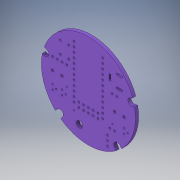
# Autodesk Inventor part: PCB
Saved by Autodesk Inventor 2018 (Build 220112000, 112)
## iProperties
Created: 2017-04-09
Part Number: PCB
Material: Fiberglass Batt
Document SubType Name: Modeling
Designer: dktur
Density: 0.032 g/cm^3
Appearance: Violet
Author: dktur
Autodesk Inventor part; units mm, degrees
ref_plane "YZ Plane" through (0, 0, 0) normal (1, 0, 0) x (0, 1, 0)
ref_plane "XZ Plane" through (0, 0, 0) normal (0, 1, 0) x (-1, 0, 0)
ref_plane "XY Plane" through (0, 0, 0) normal (0, 0, 1) x (1, 0, 0)
sketch "Sketch1" plane through (0, 0, 0) normal (0, 0, 1) x (1, 0, 0)
  arc A0 (14.5033, 41.5512) -> (15.7358, 44.915) centre (15.225, 43.1944) ccw
  line L0 (15.7358, 44.915) -> (14.5707, 45.3269)
  line L1 (14.5033, 41.5512) -> (13.575, 41.9589)
  arc A1 (24.2884, 17.9351) -> (21.5624, 20.3195) centre (22.9253, 19.1272) ccw
  line L2 (21.5624, 20.3195) -> (20.4482, 19.1255)
  line L3 (24.2884, 17.9351) -> (23.3266, 16.7167)
  arc A2 (60.3359, 44.8761) -> (61.4886, 41.4217) centre (60.8858, 43.1401) ccw
  line L4 (60.3359, 44.8761) -> (61.599, 45.4156)
  line L5 (61.4886, 41.4217) -> (62.5849, 41.742)
  arc A3 (54.5374, 20.4215) -> (51.9475, 17.877) centre (53.3634, 19.0261) ccw
  line L6 (51.9475, 17.877) -> (52.8261, 16.6745)
  line L7 (54.5374, 20.4215) -> (55.7157, 19.0618)
  arc A4 (61.599, 45.4156) -> (14.5707, 45.3269) centre (38.1009, 36.8543) ccw
  arc A5 (55.7157, 19.0618) -> (62.5849, 41.742) centre (38.1082, 36.775) ccw
  arc A6 (23.3266, 16.7167) -> (52.8261, 16.6745) centre (38.1052, 36.8421) ccw
  arc A7 (13.575, 41.9589) -> (20.4482, 19.1255) centre (38.0481, 36.8745) ccw
  circle A8 centre (33.274, 19.05) radius 1.651
  circle A9 centre (52.07, 34.29) radius 0.65
  circle A10 centre (57.07, 34.29) radius 0.65
  circle A11 centre (48.26, 19.05) radius 0.508
  circle A12 centre (48.26, 16.51) radius 0.508
  circle A13 centre (48.26, 21.59) radius 0.508
  circle A14 centre (52.07, 25.4) radius 0.508
  circle A15 centre (49.53, 25.4) radius 0.508
  circle A16 centre (45.72, 48.26) radius 0.508
  circle A17 centre (45.72, 50.8) radius 0.508
  circle A18 centre (45.72, 53.34) radius 0.508
  circle A19 centre (45.72, 55.88) radius 0.508
  circle A20 centre (19.05, 30.48) radius 0.4064
  circle A21 centre (20.955, 29.21) radius 0.4064
  circle A22 centre (19.05, 27.94) radius 0.4064
  circle A23 centre (19.05, 36.83) radius 0.65
  circle A24 centre (24.05, 36.83) radius 0.65
  circle A25 centre (30.48, 24.13) radius 0.3
  circle A26 centre (50.8, 27.94) radius 0.3
  circle A27 centre (26.67, 33.02) radius 0.3
  circle A28 centre (54.57, 52.19) radius 0.5
  circle A29 centre (49.57, 48.89) radius 0.5
  circle A30 centre (54.57, 45.89) radius 0.5
  circle A31 centre (53.34, 41.91) radius 0.508
  circle A32 centre (50.8, 41.91) radius 0.508
  circle A33 centre (33.02, 29.21) radius 0.508
  circle A34 centre (57.15, 29.21) radius 0.4064
  circle A35 centre (59.055, 27.94) radius 0.4064
  circle A36 centre (57.15, 26.67) radius 0.4064
  circle A37 centre (19.05, 43.18) radius 0.508
  circle A38 centre (21.59, 43.18) radius 0.508
  circle A39 centre (24.13, 43.18) radius 0.508
  circle A40 centre (26.67, 43.18) radius 0.508
  circle A41 centre (24.13, 30.48) radius 0.4064
  circle A42 centre (26.035, 29.21) radius 0.4064
  circle A43 centre (24.13, 27.94) radius 0.4064
  circle A44 centre (27.6606, 46.2788) radius 0.508
  circle A45 centre (27.6606, 52.7812) radius 0.508
  circle A46 centre (23.1394, 46.2788) radius 0.508
  circle A47 centre (23.1394, 52.7812) radius 0.508
  circle A48 centre (30.48, 55.88) radius 0.508
  circle A49 centre (30.48, 53.34) radius 0.508
  circle A50 centre (30.48, 50.8) radius 0.508
  circle A51 centre (30.48, 48.26) radius 0.508
  circle A52 centre (30.48, 45.72) radius 0.508
  circle A53 centre (30.48, 43.18) radius 0.508
  circle A54 centre (30.48, 40.64) radius 0.508
  circle A55 centre (30.48, 38.1) radius 0.508
  circle A56 centre (30.48, 35.56) radius 0.508
  circle A57 centre (30.48, 33.02) radius 0.508
  circle A58 centre (30.48, 30.48) radius 0.508
  circle A59 centre (30.48, 27.94) radius 0.508
  circle A60 centre (45.72, 27.94) radius 0.508
  circle A61 centre (45.72, 30.48) radius 0.508
  circle A62 centre (45.72, 33.02) radius 0.508
  circle A63 centre (45.72, 35.56) radius 0.508
  circle A64 centre (45.72, 38.1) radius 0.508
  circle A65 centre (45.72, 40.64) radius 0.508
  circle A66 centre (45.72, 43.18) radius 0.508
  circle A67 centre (45.72, 45.72) radius 0.508
  line L8 (56.17, 45.89) -> (52.97, 45.89)
  arc A68 (55.67, 45.39) -> (56.17, 45.89) centre (55.67, 45.89) ccw
  line L9 (55.67, 45.39) -> (53.47, 45.39)
  arc A69 (52.97, 45.89) -> (53.47, 45.39) centre (53.47, 45.89) ccw
  arc A70 (53.47, 46.39) -> (52.97, 45.89) centre (53.47, 45.89) ccw
  line L10 (53.47, 46.39) -> (55.67, 46.39)
  arc A71 (56.17, 45.89) -> (55.67, 46.39) centre (55.67, 45.89) ccw
  arc A72 (55.67, 51.69) -> (56.17, 52.19) centre (55.67, 52.19) ccw
  line L11 (55.67, 51.69) -> (53.47, 51.69)
  arc A73 (52.97, 52.19) -> (53.47, 51.69) centre (53.47, 52.19) ccw
  arc A74 (53.47, 52.69) -> (52.97, 52.19) centre (53.47, 52.19) ccw
  line L12 (53.47, 52.69) -> (55.67, 52.69)
  arc A75 (49.57, 47.29) -> (50.07, 47.79) centre (49.57, 47.79) ccw
  arc A76 (49.07, 47.79) -> (49.57, 47.29) centre (49.57, 47.79) ccw
  line L13 (49.07, 47.79) -> (49.07, 49.99)
  arc A77 (49.57, 50.49) -> (49.07, 49.99) centre (49.57, 49.99) ccw
  arc A78 (50.07, 49.99) -> (49.57, 50.49) centre (49.57, 49.99) ccw
  arc A79 (56.17, 52.19) -> (55.67, 52.69) centre (55.67, 52.19) ccw
  line L14 (50.07, 49.99) -> (50.07, 47.79)
  arc A80 (57.07, 33.782) -> (57.07, 34.798) centre (57.07, 34.29) ccw
  arc A81 (57.07, 34.798) -> (57.07, 33.782) centre (57.07, 34.29) ccw
  arc A82 (57.07, 33.782) -> (57.07, 34.798) centre (57.07, 34.29) ccw
  arc A83 (57.07, 34.798) -> (57.07, 33.782) centre (57.07, 34.29) ccw
  line L15 (49.022, 19.05) -> (47.498, 19.05)
  arc A84 (47.498, 19.431) -> (47.498, 18.669) centre (47.498, 19.05) ccw
  arc A85 (49.022, 18.669) -> (49.022, 19.431) centre (49.022, 19.05) ccw
  line L16 (49.022, 19.05) -> (47.498, 19.05)
  arc A86 (47.498, 19.431) -> (47.498, 18.669) centre (47.498, 19.05) ccw
  arc A87 (49.022, 18.669) -> (49.022, 19.431) centre (49.022, 19.05) ccw
  line L17 (49.022, 16.51) -> (47.498, 16.51)
  arc A88 (47.498, 16.891) -> (47.498, 16.129) centre (47.498, 16.51) ccw
  arc A89 (49.022, 16.129) -> (49.022, 16.891) centre (49.022, 16.51) ccw
  line L18 (49.022, 16.51) -> (47.498, 16.51)
  arc A90 (47.498, 16.891) -> (47.498, 16.129) centre (47.498, 16.51) ccw
  arc A91 (49.022, 16.129) -> (49.022, 16.891) centre (49.022, 16.51) ccw
  line L19 (49.022, 21.59) -> (47.498, 21.59)
  arc A92 (47.498, 21.971) -> (47.498, 21.209) centre (47.498, 21.59) ccw
  arc A93 (49.022, 21.209) -> (49.022, 21.971) centre (49.022, 21.59) ccw
  line L20 (49.022, 21.59) -> (47.498, 21.59)
  arc A94 (47.498, 21.971) -> (47.498, 21.209) centre (47.498, 21.59) ccw
  arc A95 (49.022, 21.209) -> (49.022, 21.971) centre (49.022, 21.59) ccw
  arc A96 (51.6001, 25.4) -> (52.5399, 25.4) centre (52.07, 25.4) ccw
  arc A97 (52.5399, 25.4) -> (51.6001, 25.4) centre (52.07, 25.4) ccw
  arc A98 (51.6001, 25.4) -> (52.5399, 25.4) centre (52.07, 25.4) ccw
  arc A99 (52.5399, 25.4) -> (51.6001, 25.4) centre (52.07, 25.4) ccw
  arc A100 (49.0601, 25.4) -> (49.9999, 25.4) centre (49.53, 25.4) ccw
  arc A101 (49.9999, 25.4) -> (49.0601, 25.4) centre (49.53, 25.4) ccw
  arc A102 (49.0601, 25.4) -> (49.9999, 25.4) centre (49.53, 25.4) ccw
  arc A103 (49.9999, 25.4) -> (49.0601, 25.4) centre (49.53, 25.4) ccw
  line L21 (55.57, 52.19) -> (53.57, 52.19)
  arc A104 (53.57, 52.69) -> (53.57, 51.69) centre (53.57, 52.19) ccw
  arc A105 (55.57, 51.69) -> (55.57, 52.69) centre (55.57, 52.19) ccw
  line L22 (55.57, 52.19) -> (53.57, 52.19)
  arc A106 (53.57, 52.69) -> (53.57, 51.69) centre (53.57, 52.19) ccw
  arc A107 (55.57, 51.69) -> (55.57, 52.69) centre (55.57, 52.19) ccw
  line L23 (49.57, 49.89) -> (49.57, 47.89)
  arc A108 (49.07, 47.89) -> (50.07, 47.89) centre (49.57, 47.89) ccw
  arc A109 (50.07, 49.89) -> (49.07, 49.89) centre (49.57, 49.89) ccw
  line L24 (49.57, 49.89) -> (49.57, 47.89)
  arc A110 (49.07, 47.89) -> (50.07, 47.89) centre (49.57, 47.89) ccw
  arc A111 (50.07, 49.89) -> (49.07, 49.89) centre (49.57, 49.89) ccw
  line L25 (55.57, 45.89) -> (53.57, 45.89)
  arc A112 (53.57, 46.39) -> (53.57, 45.39) centre (53.57, 45.89) ccw
  arc A113 (55.57, 45.39) -> (55.57, 46.39) centre (55.57, 45.89) ccw
  line L26 (55.57, 45.89) -> (53.57, 45.89)
  arc A114 (53.57, 46.39) -> (53.57, 45.39) centre (53.57, 45.89) ccw
  arc A115 (55.57, 45.39) -> (55.57, 46.39) centre (55.57, 45.89) ccw
  arc A116 (52.8701, 41.91) -> (53.8099, 41.91) centre (53.34, 41.91) ccw
  arc A117 (53.8099, 41.91) -> (52.8701, 41.91) centre (53.34, 41.91) ccw
  arc A118 (52.8701, 41.91) -> (53.8099, 41.91) centre (53.34, 41.91) ccw
  arc A119 (53.8099, 41.91) -> (52.8701, 41.91) centre (53.34, 41.91) ccw
  arc A120 (50.3301, 41.91) -> (51.2699, 41.91) centre (50.8, 41.91) ccw
  arc A121 (51.2699, 41.91) -> (50.3301, 41.91) centre (50.8, 41.91) ccw
  arc A122 (50.3301, 41.91) -> (51.2699, 41.91) centre (50.8, 41.91) ccw
  arc A123 (51.2699, 41.91) -> (50.3301, 41.91) centre (50.8, 41.91) ccw
  line L27 (57.2763, 28.9052) -> (57.0237, 28.9052)
  line L28 (57.0237, 28.9052) -> (56.8452, 29.0837)
  line L29 (56.8452, 29.0837) -> (56.8452, 29.3363)
  line L30 (56.8452, 29.3363) -> (57.0237, 29.5148)
  line L31 (57.0237, 29.5148) -> (57.2763, 29.5148)
  line L32 (57.2763, 29.5148) -> (57.4548, 29.3363)
  line L33 (57.4548, 29.3363) -> (57.4548, 29.0837)
  line L34 (57.4548, 29.0837) -> (57.2763, 28.9052)
  line L35 (57.2763, 28.9052) -> (57.0237, 28.9052)
  line L36 (57.2763, 28.9052) -> (57.0237, 28.9052)
  line L37 (57.0237, 28.9052) -> (56.8452, 29.0837)
  line L38 (56.8452, 29.0837) -> (56.8452, 29.3363)
  line L39 (56.8452, 29.3363) -> (57.0237, 29.5148)
  line L40 (57.0237, 29.5148) -> (57.2763, 29.5148)
  line L41 (57.2763, 29.5148) -> (57.4548, 29.3363)
  line L42 (57.4548, 29.3363) -> (57.4548, 29.0837)
  line L43 (57.4548, 29.0837) -> (57.2763, 28.9052)
  line L44 (57.2763, 28.9052) -> (57.0237, 28.9052)
  line L45 (59.1813, 27.6352) -> (58.9287, 27.6352)
  line L46 (58.9287, 27.6352) -> (58.7502, 27.8137)
  line L47 (58.7502, 27.8137) -> (58.7502, 28.0663)
  line L48 (58.7502, 28.0663) -> (58.9287, 28.2448)
  line L49 (58.9287, 28.2448) -> (59.1813, 28.2448)
  line L50 (59.1813, 28.2448) -> (59.3598, 28.0663)
  line L51 (59.3598, 28.0663) -> (59.3598, 27.8137)
  line L52 (59.3598, 27.8137) -> (59.1813, 27.6352)
  line L53 (59.1813, 27.6352) -> (58.9287, 27.6352)
  line L54 (59.1813, 27.6352) -> (58.9287, 27.6352)
  line L55 (58.9287, 27.6352) -> (58.7502, 27.8137)
  line L56 (58.7502, 27.8137) -> (58.7502, 28.0663)
  line L57 (58.7502, 28.0663) -> (58.9287, 28.2448)
  line L58 (58.9287, 28.2448) -> (59.1813, 28.2448)
  line L59 (59.1813, 28.2448) -> (59.3598, 28.0663)
  line L60 (59.3598, 28.0663) -> (59.3598, 27.8137)
  line L61 (59.3598, 27.8137) -> (59.1813, 27.6352)
  line L62 (59.1813, 27.6352) -> (58.9287, 27.6352)
  line L63 (57.2763, 26.3652) -> (57.0237, 26.3652)
  line L64 (57.0237, 26.3652) -> (56.8452, 26.5437)
  line L65 (56.8452, 26.5437) -> (56.8452, 26.7963)
  line L66 (56.8452, 26.7963) -> (57.0237, 26.9748)
  line L67 (57.0237, 26.9748) -> (57.2763, 26.9748)
  line L68 (57.2763, 26.9748) -> (57.4548, 26.7963)
  line L69 (57.4548, 26.7963) -> (57.4548, 26.5437)
  line L70 (57.4548, 26.5437) -> (57.2763, 26.3652)
  line L71 (57.2763, 26.3652) -> (57.0237, 26.3652)
  line L72 (57.2763, 26.3652) -> (57.0237, 26.3652)
  line L73 (57.0237, 26.3652) -> (56.8452, 26.5437)
  line L74 (56.8452, 26.5437) -> (56.8452, 26.7963)
  line L75 (56.8452, 26.7963) -> (57.0237, 26.9748)
  line L76 (57.0237, 26.9748) -> (57.2763, 26.9748)
  line L77 (57.2763, 26.9748) -> (57.4548, 26.7963)
  line L78 (57.4548, 26.7963) -> (57.4548, 26.5437)
  line L79 (57.4548, 26.5437) -> (57.2763, 26.3652)
  line L80 (57.2763, 26.3652) -> (57.0237, 26.3652)
  arc A124 (19.5199, 43.18) -> (18.5801, 43.18) centre (19.05, 43.18) ccw
  arc A125 (18.5801, 43.18) -> (19.5199, 43.18) centre (19.05, 43.18) ccw
  arc A126 (19.5199, 43.18) -> (18.5801, 43.18) centre (19.05, 43.18) ccw
  arc A127 (18.5801, 43.18) -> (19.5199, 43.18) centre (19.05, 43.18) ccw
  arc A128 (22.0599, 43.18) -> (21.1201, 43.18) centre (21.59, 43.18) ccw
  arc A129 (21.1201, 43.18) -> (22.0599, 43.18) centre (21.59, 43.18) ccw
  arc A130 (22.0599, 43.18) -> (21.1201, 43.18) centre (21.59, 43.18) ccw
  arc A131 (21.1201, 43.18) -> (22.0599, 43.18) centre (21.59, 43.18) ccw
  arc A132 (24.5999, 43.18) -> (23.6601, 43.18) centre (24.13, 43.18) ccw
  arc A133 (23.6601, 43.18) -> (24.5999, 43.18) centre (24.13, 43.18) ccw
  arc A134 (24.5999, 43.18) -> (23.6601, 43.18) centre (24.13, 43.18) ccw
  arc A135 (23.6601, 43.18) -> (24.5999, 43.18) centre (24.13, 43.18) ccw
  arc A136 (27.1399, 43.18) -> (26.2001, 43.18) centre (26.67, 43.18) ccw
  arc A137 (26.2001, 43.18) -> (27.1399, 43.18) centre (26.67, 43.18) ccw
  arc A138 (27.1399, 43.18) -> (26.2001, 43.18) centre (26.67, 43.18) ccw
  arc A139 (26.2001, 43.18) -> (27.1399, 43.18) centre (26.67, 43.18) ccw
  line L81 (24.2563, 30.1752) -> (24.0037, 30.1752)
  line L82 (24.0037, 30.1752) -> (23.8252, 30.3537)
  line L83 (23.8252, 30.3537) -> (23.8252, 30.6063)
  line L84 (23.8252, 30.6063) -> (24.0037, 30.7848)
  line L85 (24.0037, 30.7848) -> (24.2563, 30.7848)
  line L86 (24.2563, 30.7848) -> (24.4348, 30.6063)
  line L87 (24.4348, 30.6063) -> (24.4348, 30.3537)
  line L88 (24.4348, 30.3537) -> (24.2563, 30.1752)
  line L89 (24.2563, 30.1752) -> (24.0037, 30.1752)
  line L90 (24.2563, 30.1752) -> (24.0037, 30.1752)
  line L91 (24.0037, 30.1752) -> (23.8252, 30.3537)
  line L92 (23.8252, 30.3537) -> (23.8252, 30.6063)
  line L93 (23.8252, 30.6063) -> (24.0037, 30.7848)
  line L94 (24.0037, 30.7848) -> (24.2563, 30.7848)
  line L95 (24.2563, 30.7848) -> (24.4348, 30.6063)
  line L96 (24.4348, 30.6063) -> (24.4348, 30.3537)
  line L97 (24.4348, 30.3537) -> (24.2563, 30.1752)
  line L98 (24.2563, 30.1752) -> (24.0037, 30.1752)
  line L99 (26.1613, 28.9052) -> (25.9087, 28.9052)
  line L100 (25.9087, 28.9052) -> (25.7302, 29.0837)
  line L101 (25.7302, 29.0837) -> (25.7302, 29.3363)
  line L102 (25.7302, 29.3363) -> (25.9087, 29.5148)
  line L103 (25.9087, 29.5148) -> (26.1613, 29.5148)
  line L104 (26.1613, 29.5148) -> (26.3398, 29.3363)
  line L105 (26.3398, 29.3363) -> (26.3398, 29.0837)
  line L106 (26.3398, 29.0837) -> (26.1613, 28.9052)
  line L107 (26.1613, 28.9052) -> (25.9087, 28.9052)
  line L108 (26.1613, 28.9052) -> (25.9087, 28.9052)
  line L109 (25.9087, 28.9052) -> (25.7302, 29.0837)
  line L110 (25.7302, 29.0837) -> (25.7302, 29.3363)
  line L111 (25.7302, 29.3363) -> (25.9087, 29.5148)
  line L112 (25.9087, 29.5148) -> (26.1613, 29.5148)
  line L113 (26.1613, 29.5148) -> (26.3398, 29.3363)
  line L114 (26.3398, 29.3363) -> (26.3398, 29.0837)
  line L115 (26.3398, 29.0837) -> (26.1613, 28.9052)
  line L116 (26.1613, 28.9052) -> (25.9087, 28.9052)
  line L117 (24.2563, 27.6352) -> (24.0037, 27.6352)
  line L118 (24.0037, 27.6352) -> (23.8252, 27.8137)
  line L119 (23.8252, 27.8137) -> (23.8252, 28.0663)
  line L120 (23.8252, 28.0663) -> (24.0037, 28.2448)
  line L121 (24.0037, 28.2448) -> (24.2563, 28.2448)
  line L122 (24.2563, 28.2448) -> (24.4348, 28.0663)
  line L123 (24.4348, 28.0663) -> (24.4348, 27.8137)
  line L124 (24.4348, 27.8137) -> (24.2563, 27.6352)
  line L125 (24.2563, 27.6352) -> (24.0037, 27.6352)
  line L126 (24.2563, 27.6352) -> (24.0037, 27.6352)
  line L127 (24.0037, 27.6352) -> (23.8252, 27.8137)
  line L128 (23.8252, 27.8137) -> (23.8252, 28.0663)
  line L129 (23.8252, 28.0663) -> (24.0037, 28.2448)
  line L130 (24.0037, 28.2448) -> (24.2563, 28.2448)
  line L131 (24.2563, 28.2448) -> (24.4348, 28.0663)
  line L132 (24.4348, 28.0663) -> (24.4348, 27.8137)
  line L133 (24.4348, 27.8137) -> (24.2563, 27.6352)
  line L134 (24.2563, 27.6352) -> (24.0037, 27.6352)
  arc A140 (28.1305, 46.2788) -> (27.1907, 46.2788) centre (27.6606, 46.2788) ccw
  arc A141 (27.1907, 46.2788) -> (28.1305, 46.2788) centre (27.6606, 46.2788) ccw
  arc A142 (28.1305, 46.2788) -> (27.1907, 46.2788) centre (27.6606, 46.2788) ccw
  arc A143 (27.1907, 46.2788) -> (28.1305, 46.2788) centre (27.6606, 46.2788) ccw
  arc A144 (28.1305, 52.7812) -> (27.1907, 52.7812) centre (27.6606, 52.7812) ccw
  arc A145 (27.1907, 52.7812) -> (28.1305, 52.7812) centre (27.6606, 52.7812) ccw
  arc A146 (28.1305, 52.7812) -> (27.1907, 52.7812) centre (27.6606, 52.7812) ccw
  arc A147 (27.1907, 52.7812) -> (28.1305, 52.7812) centre (27.6606, 52.7812) ccw
  arc A148 (23.6093, 46.2788) -> (22.6695, 46.2788) centre (23.1394, 46.2788) ccw
  arc A149 (22.6695, 46.2788) -> (23.6093, 46.2788) centre (23.1394, 46.2788) ccw
  arc A150 (23.6093, 46.2788) -> (22.6695, 46.2788) centre (23.1394, 46.2788) ccw
  arc A151 (22.6695, 46.2788) -> (23.6093, 46.2788) centre (23.1394, 46.2788) ccw
  arc A152 (23.6093, 52.7812) -> (22.6695, 52.7812) centre (23.1394, 52.7812) ccw
  arc A153 (22.6695, 52.7812) -> (23.6093, 52.7812) centre (23.1394, 52.7812) ccw
  arc A154 (23.6093, 52.7812) -> (22.6695, 52.7812) centre (23.1394, 52.7812) ccw
  arc A155 (22.6695, 52.7812) -> (23.6093, 52.7812) centre (23.1394, 52.7812) ccw
  arc A156 (30.48, 55.4101) -> (30.48, 56.3499) centre (30.48, 55.88) ccw
  arc A157 (30.48, 56.3499) -> (30.48, 55.4101) centre (30.48, 55.88) ccw
  arc A158 (30.48, 55.4101) -> (30.48, 56.3499) centre (30.48, 55.88) ccw
  arc A159 (30.48, 56.3499) -> (30.48, 55.4101) centre (30.48, 55.88) ccw
  arc A160 (30.48, 52.8701) -> (30.48, 53.8099) centre (30.48, 53.34) ccw
  arc A161 (30.48, 53.8099) -> (30.48, 52.8701) centre (30.48, 53.34) ccw
  arc A162 (30.48, 52.8701) -> (30.48, 53.8099) centre (30.48, 53.34) ccw
  arc A163 (30.48, 53.8099) -> (30.48, 52.8701) centre (30.48, 53.34) ccw
  arc A164 (30.48, 50.3301) -> (30.48, 51.2699) centre (30.48, 50.8) ccw
  arc A165 (30.48, 51.2699) -> (30.48, 50.3301) centre (30.48, 50.8) ccw
  arc A166 (30.48, 50.3301) -> (30.48, 51.2699) centre (30.48, 50.8) ccw
  arc A167 (30.48, 51.2699) -> (30.48, 50.3301) centre (30.48, 50.8) ccw
  arc A168 (30.48, 47.7901) -> (30.48, 48.7299) centre (30.48, 48.26) ccw
  arc A169 (30.48, 48.7299) -> (30.48, 47.7901) centre (30.48, 48.26) ccw
  arc A170 (30.48, 47.7901) -> (30.48, 48.7299) centre (30.48, 48.26) ccw
  arc A171 (30.48, 48.7299) -> (30.48, 47.7901) centre (30.48, 48.26) ccw
  arc A172 (30.48, 45.2501) -> (30.48, 46.1899) centre (30.48, 45.72) ccw
  arc A173 (30.48, 46.1899) -> (30.48, 45.2501) centre (30.48, 45.72) ccw
  arc A174 (30.48, 45.2501) -> (30.48, 46.1899) centre (30.48, 45.72) ccw
  arc A175 (30.48, 46.1899) -> (30.48, 45.2501) centre (30.48, 45.72) ccw
  arc A176 (30.48, 42.7101) -> (30.48, 43.6499) centre (30.48, 43.18) ccw
  arc A177 (30.48, 43.6499) -> (30.48, 42.7101) centre (30.48, 43.18) ccw
  arc A178 (30.48, 42.7101) -> (30.48, 43.6499) centre (30.48, 43.18) ccw
  arc A179 (30.48, 43.6499) -> (30.48, 42.7101) centre (30.48, 43.18) ccw
  arc A180 (30.48, 40.1701) -> (30.48, 41.1099) centre (30.48, 40.64) ccw
  arc A181 (30.48, 41.1099) -> (30.48, 40.1701) centre (30.48, 40.64) ccw
  arc A182 (30.48, 40.1701) -> (30.48, 41.1099) centre (30.48, 40.64) ccw
  arc A183 (30.48, 41.1099) -> (30.48, 40.1701) centre (30.48, 40.64) ccw
  arc A184 (30.48, 37.6301) -> (30.48, 38.5699) centre (30.48, 38.1) ccw
  arc A185 (30.48, 38.5699) -> (30.48, 37.6301) centre (30.48, 38.1) ccw
  arc A186 (30.48, 37.6301) -> (30.48, 38.5699) centre (30.48, 38.1) ccw
  arc A187 (30.48, 38.5699) -> (30.48, 37.6301) centre (30.48, 38.1) ccw
  arc A188 (30.48, 35.0901) -> (30.48, 36.0299) centre (30.48, 35.56) ccw
  arc A189 (30.48, 36.0299) -> (30.48, 35.0901) centre (30.48, 35.56) ccw
  arc A190 (30.48, 35.0901) -> (30.48, 36.0299) centre (30.48, 35.56) ccw
  arc A191 (30.48, 36.0299) -> (30.48, 35.0901) centre (30.48, 35.56) ccw
  arc A192 (30.48, 32.5501) -> (30.48, 33.4899) centre (30.48, 33.02) ccw
  arc A193 (30.48, 33.4899) -> (30.48, 32.5501) centre (30.48, 33.02) ccw
  arc A194 (30.48, 32.5501) -> (30.48, 33.4899) centre (30.48, 33.02) ccw
  arc A195 (30.48, 33.4899) -> (30.48, 32.5501) centre (30.48, 33.02) ccw
  arc A196 (30.48, 30.0101) -> (30.48, 30.9499) centre (30.48, 30.48) ccw
  arc A197 (30.48, 30.9499) -> (30.48, 30.0101) centre (30.48, 30.48) ccw
  arc A198 (30.48, 30.0101) -> (30.48, 30.9499) centre (30.48, 30.48) ccw
  arc A199 (30.48, 30.9499) -> (30.48, 30.0101) centre (30.48, 30.48) ccw
  arc A200 (30.48, 27.4701) -> (30.48, 28.4099) centre (30.48, 27.94) ccw
  arc A201 (30.48, 28.4099) -> (30.48, 27.4701) centre (30.48, 27.94) ccw
  arc A202 (30.48, 27.4701) -> (30.48, 28.4099) centre (30.48, 27.94) ccw
  arc A203 (30.48, 28.4099) -> (30.48, 27.4701) centre (30.48, 27.94) ccw
  arc A204 (45.72, 27.4701) -> (45.72, 28.4099) centre (45.72, 27.94) ccw
  arc A205 (45.72, 28.4099) -> (45.72, 27.4701) centre (45.72, 27.94) ccw
  arc A206 (45.72, 27.4701) -> (45.72, 28.4099) centre (45.72, 27.94) ccw
  arc A207 (45.72, 28.4099) -> (45.72, 27.4701) centre (45.72, 27.94) ccw
  arc A208 (45.72, 30.0101) -> (45.72, 30.9499) centre (45.72, 30.48) ccw
  arc A209 (45.72, 30.9499) -> (45.72, 30.0101) centre (45.72, 30.48) ccw
  arc A210 (45.72, 30.0101) -> (45.72, 30.9499) centre (45.72, 30.48) ccw
  arc A211 (45.72, 30.9499) -> (45.72, 30.0101) centre (45.72, 30.48) ccw
  arc A212 (45.72, 32.5501) -> (45.72, 33.4899) centre (45.72, 33.02) ccw
  arc A213 (45.72, 33.4899) -> (45.72, 32.5501) centre (45.72, 33.02) ccw
  arc A214 (45.72, 32.5501) -> (45.72, 33.4899) centre (45.72, 33.02) ccw
  arc A215 (45.72, 33.4899) -> (45.72, 32.5501) centre (45.72, 33.02) ccw
  arc A216 (45.72, 35.0901) -> (45.72, 36.0299) centre (45.72, 35.56) ccw
  arc A217 (45.72, 36.0299) -> (45.72, 35.0901) centre (45.72, 35.56) ccw
  arc A218 (45.72, 35.0901) -> (45.72, 36.0299) centre (45.72, 35.56) ccw
  arc A219 (45.72, 36.0299) -> (45.72, 35.0901) centre (45.72, 35.56) ccw
  arc A220 (45.72, 37.6301) -> (45.72, 38.5699) centre (45.72, 38.1) ccw
  arc A221 (45.72, 38.5699) -> (45.72, 37.6301) centre (45.72, 38.1) ccw
  arc A222 (45.72, 37.6301) -> (45.72, 38.5699) centre (45.72, 38.1) ccw
  arc A223 (45.72, 38.5699) -> (45.72, 37.6301) centre (45.72, 38.1) ccw
  arc A224 (45.72, 40.1701) -> (45.72, 41.1099) centre (45.72, 40.64) ccw
  arc A225 (45.72, 41.1099) -> (45.72, 40.1701) centre (45.72, 40.64) ccw
  arc A226 (45.72, 40.1701) -> (45.72, 41.1099) centre (45.72, 40.64) ccw
  arc A227 (45.72, 41.1099) -> (45.72, 40.1701) centre (45.72, 40.64) ccw
  arc A228 (45.72, 42.7101) -> (45.72, 43.6499) centre (45.72, 43.18) ccw
  arc A229 (45.72, 43.6499) -> (45.72, 42.7101) centre (45.72, 43.18) ccw
  arc A230 (45.72, 42.7101) -> (45.72, 43.6499) centre (45.72, 43.18) ccw
  arc A231 (45.72, 43.6499) -> (45.72, 42.7101) centre (45.72, 43.18) ccw
  arc A232 (45.72, 45.2501) -> (45.72, 46.1899) centre (45.72, 45.72) ccw
  arc A233 (45.72, 46.1899) -> (45.72, 45.2501) centre (45.72, 45.72) ccw
  arc A234 (45.72, 45.2501) -> (45.72, 46.1899) centre (45.72, 45.72) ccw
  arc A235 (45.72, 46.1899) -> (45.72, 45.2501) centre (45.72, 45.72) ccw
  arc A236 (45.72, 47.7901) -> (45.72, 48.7299) centre (45.72, 48.26) ccw
  arc A237 (45.72, 48.7299) -> (45.72, 47.7901) centre (45.72, 48.26) ccw
  arc A238 (45.72, 47.7901) -> (45.72, 48.7299) centre (45.72, 48.26) ccw
  arc A239 (45.72, 48.7299) -> (45.72, 47.7901) centre (45.72, 48.26) ccw
  arc A240 (45.72, 50.3301) -> (45.72, 51.2699) centre (45.72, 50.8) ccw
  arc A241 (45.72, 51.2699) -> (45.72, 50.3301) centre (45.72, 50.8) ccw
  arc A242 (45.72, 50.3301) -> (45.72, 51.2699) centre (45.72, 50.8) ccw
  arc A243 (45.72, 51.2699) -> (45.72, 50.3301) centre (45.72, 50.8) ccw
  arc A244 (45.72, 52.8701) -> (45.72, 53.8099) centre (45.72, 53.34) ccw
  arc A245 (45.72, 53.8099) -> (45.72, 52.8701) centre (45.72, 53.34) ccw
  arc A246 (45.72, 52.8701) -> (45.72, 53.8099) centre (45.72, 53.34) ccw
  arc A247 (45.72, 53.8099) -> (45.72, 52.8701) centre (45.72, 53.34) ccw
  arc A248 (45.72, 55.4101) -> (45.72, 56.3499) centre (45.72, 55.88) ccw
  arc A249 (45.72, 56.3499) -> (45.72, 55.4101) centre (45.72, 55.88) ccw
  arc A250 (45.72, 55.4101) -> (45.72, 56.3499) centre (45.72, 55.88) ccw
  arc A251 (45.72, 56.3499) -> (45.72, 55.4101) centre (45.72, 55.88) ccw
  line L135 (19.1763, 30.1752) -> (18.9237, 30.1752)
  line L136 (18.9237, 30.1752) -> (18.7452, 30.3537)
  line L137 (18.7452, 30.3537) -> (18.7452, 30.6063)
  line L138 (18.7452, 30.6063) -> (18.9237, 30.7848)
  line L139 (18.9237, 30.7848) -> (19.1763, 30.7848)
  line L140 (19.1763, 30.7848) -> (19.3548, 30.6063)
  line L141 (19.3548, 30.6063) -> (19.3548, 30.3537)
  line L142 (19.3548, 30.3537) -> (19.1763, 30.1752)
  line L143 (19.1763, 30.1752) -> (18.9237, 30.1752)
  line L144 (19.1763, 30.1752) -> (18.9237, 30.1752)
  line L145 (18.9237, 30.1752) -> (18.7452, 30.3537)
  line L146 (18.7452, 30.3537) -> (18.7452, 30.6063)
  line L147 (18.7452, 30.6063) -> (18.9237, 30.7848)
  line L148 (18.9237, 30.7848) -> (19.1763, 30.7848)
  line L149 (19.1763, 30.7848) -> (19.3548, 30.6063)
  line L150 (19.3548, 30.6063) -> (19.3548, 30.3537)
  line L151 (19.3548, 30.3537) -> (19.1763, 30.1752)
  line L152 (19.1763, 30.1752) -> (18.9237, 30.1752)
  line L153 (21.0813, 28.9052) -> (20.8287, 28.9052)
  line L154 (20.8287, 28.9052) -> (20.6502, 29.0837)
  line L155 (20.6502, 29.0837) -> (20.6502, 29.3363)
  line L156 (20.6502, 29.3363) -> (20.8287, 29.5148)
  line L157 (20.8287, 29.5148) -> (21.0813, 29.5148)
  line L158 (21.0813, 29.5148) -> (21.2598, 29.3363)
  line L159 (21.2598, 29.3363) -> (21.2598, 29.0837)
  line L160 (21.2598, 29.0837) -> (21.0813, 28.9052)
  line L161 (21.0813, 28.9052) -> (20.8287, 28.9052)
  line L162 (21.0813, 28.9052) -> (20.8287, 28.9052)
  line L163 (20.8287, 28.9052) -> (20.6502, 29.0837)
  line L164 (20.6502, 29.0837) -> (20.6502, 29.3363)
  line L165 (20.6502, 29.3363) -> (20.8287, 29.5148)
  line L166 (20.8287, 29.5148) -> (21.0813, 29.5148)
  line L167 (21.0813, 29.5148) -> (21.2598, 29.3363)
  line L168 (21.2598, 29.3363) -> (21.2598, 29.0837)
  line L169 (21.2598, 29.0837) -> (21.0813, 28.9052)
  line L170 (21.0813, 28.9052) -> (20.8287, 28.9052)
  line L171 (19.1763, 27.6352) -> (18.9237, 27.6352)
  line L172 (18.9237, 27.6352) -> (18.7452, 27.8137)
  line L173 (18.7452, 27.8137) -> (18.7452, 28.0663)
  line L174 (18.7452, 28.0663) -> (18.9237, 28.2448)
  line L175 (18.9237, 28.2448) -> (19.1763, 28.2448)
  line L176 (19.1763, 28.2448) -> (19.3548, 28.0663)
  line L177 (19.3548, 28.0663) -> (19.3548, 27.8137)
  line L178 (19.3548, 27.8137) -> (19.1763, 27.6352)
  line L179 (19.1763, 27.6352) -> (18.9237, 27.6352)
  line L180 (19.1763, 27.6352) -> (18.9237, 27.6352)
  line L181 (18.9237, 27.6352) -> (18.7452, 27.8137)
  line L182 (18.7452, 27.8137) -> (18.7452, 28.0663)
  line L183 (18.7452, 28.0663) -> (18.9237, 28.2448)
  line L184 (18.9237, 28.2448) -> (19.1763, 28.2448)
  line L185 (19.1763, 28.2448) -> (19.3548, 28.0663)
  line L186 (19.3548, 28.0663) -> (19.3548, 27.8137)
  line L187 (19.3548, 27.8137) -> (19.1763, 27.6352)
  line L188 (19.1763, 27.6352) -> (18.9237, 27.6352)
  arc A252 (24.05, 36.322) -> (24.05, 37.338) centre (24.05, 36.83) ccw
  arc A253 (24.05, 37.338) -> (24.05, 36.322) centre (24.05, 36.83) ccw
  arc A254 (24.05, 36.322) -> (24.05, 37.338) centre (24.05, 36.83) ccw
  arc A255 (24.05, 37.338) -> (24.05, 36.322) centre (24.05, 36.83) ccw
  circle A256 centre (33.02, 29.21) radius 0.5086
  circle A257 centre (33.02, 26.67) radius 0.508
  circle A258 centre (35.56, 29.21) radius 0.508
  circle A259 centre (35.56, 26.67) radius 0.508
  circle A260 centre (38.1, 29.21) radius 0.508
  circle A261 centre (38.1, 26.67) radius 0.508
  circle A262 centre (40.64, 29.21) radius 0.508
  circle A263 centre (40.64, 26.67) radius 0.508
  circle A264 centre (43.18, 29.21) radius 0.508
  circle A265 centre (43.18, 26.67) radius 0.508
  point P0 (0, 0)
  dimension "d4" = 2.54
  dimension "d7" = 2.54
  constraints: 392 point on circle, 378 end point, 266 centre point, 74 perpendicular, 72 equal radius, 39 parallel, 7 tangent, 1 coincident, 1 horizontal, 1 vertical, 18 other
  measures "d4" distance of A33.centre A257.centre
  measures "d7" distance of A33.centre A258.centre
extrude "Extrusion2" add sketch "Sketch1" along normal blind 1.67 contours A0 L0 A4 L4 A2 L5 A5 L7 A3 L6 A6 L3 A1 L2 A7 L1
body "Solid2"
